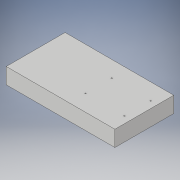
# Autodesk Inventor part: Chassis
Saved by Autodesk Inventor 2019 (Build 230136000, 136)
## iProperties
Created: 2020-02-14
Part Number: Chassis
Material: Generic
Document SubType Name: Modeling
Designer: close
Density: 1 g/cm^3
Appearance: Default
Author: close
Autodesk Inventor part; units mm, degrees
ref_plane "YZ Plane" through (0, 0, 0) normal (1, 0, 0) x (0, 1, 0)
ref_plane "XZ Plane" through (0, 0, 0) normal (0, 1, 0) x (-1, 0, 0)
ref_plane "XY Plane" through (0, 0, 0) normal (0, 0, 1) x (1, 0, 0)
sketch "Sketch1" plane through (0, 0, 0) normal (0, 1, 0) x (-1, 0, 0)
  line L0 (0, 0) -> (240, 0)
  line L1 (240, 0) -> (240, -130)
  line L2 (240, -130) -> (0, -130)
  line L3 (0, -130) -> (0, 0)
  dimension "d0" = 130
  dimension "d1" = 240
  constraints: 8 end point, 2 parallel, 1 horizontal, 1 perpendicular
  measures "d0" distance between parallel lines of L2 L0
  measures "d1" distance between parallel lines of L3 L1
extrude "Extrusion1" add sketch "Sketch1" along normal blind 35
sketch "Sketch2" plane through (0, 0, 0) normal (0, -1, 0) x (1, 0, 0)
  line L0 (-5, -111) -> (-105, -111) construction
  line L1 (-105, -111) -> (-105, -32) construction
  line L2 (-105, -32) -> (-5, -32) construction
  line L3 (-5, -32) -> (-5, -111) construction
  line L4 (-15, -94) -> (-101, -94) construction
  line L5 (-101, -94) -> (-101, -36) construction
  line L6 (-101, -36) -> (-15, -36) construction
  line L7 (-15, -36) -> (-15, -94) construction
  line L8 (-103.25, -76.2) -> (-99.35, -76.2) construction
  line L9 (-99.35, -76.2) -> (-99.35, -53.8) construction
  line L10 (-99.35, -53.8) -> (-103.25, -53.8) construction
  line L11 (-103.25, -53.8) -> (-103.25, -76.2) construction
  line L12 (0, 0) -> (-240, 0) construction
  line L13 (-240, -130) -> (0, -130) construction
  line L14 (-2.5, -113.5) -> (-107.5, -113.5)
  line L15 (-107.5, -113.5) -> (-107.5, -29.5)
  line L16 (-107.5, -29.5) -> (-2.5, -29.5)
  line L17 (-2.5, -29.5) -> (-2.5, -113.5)
  line L18 (0, -130) -> (0, 0) projected
  dimension "d5" = 100
  dimension "d6" = 86
  dimension "d7" = 58
  dimension "d8" = 79
  dimension "d9" = 4
  dimension "d10" = 4
  dimension "d12" = 22.4
  dimension "d13" = 17.8
  dimension "d14" = 130
  dimension "d16" = 53.8
  dimension "d17" = 3.9
  dimension "d18" = 1.75
  dimension "d19" = 105
  dimension "d20" = 2.5
  dimension "d21" = 84
  dimension "d22" = 2.5
  dimension "d25" = 2.5
  constraints: 32 end point, 8 parallel, 4 horizontal, 4 perpendicular
  measures "d5" distance of L0.start L0.end
  measures "d6" distance of L4.start L4.end
  measures "d7" distance of L6.end L4.start
  measures "d8" distance of L2.end L0.start
  measures "d9" distance between parallel lines of L2 L6
  measures "d10" distance between parallel lines of L1 L5
  measures "d12" distance between parallel lines of L10 L8
  measures "d13" distance from line of L5.end L10
  measures "d14" distance between parallel lines of L12 L13
  measures "d16" distance between parallel lines of L13 L8
  measures "d17" distance between parallel lines of L11 L9
  measures "d18" distance between parallel lines of L1 L11
  measures "d19" distance of L14.start L14.end
  measures "d20" distance between parallel lines of L18 L17
  measures "d21" distance between parallel lines of L16 L14
  measures "d22" distance between parallel lines of L0 L14
  measures "d25" distance between parallel lines of L17 L3
extrude "Extrusion2" cut sketch "Sketch2" against normal blind 32.5
sketch "Sketch3" plane through (0, 32.5, 0) normal (0, -1, 0) x (1, 0, 0)
  circle A0 centre (-15, -94) radius 3
  circle A1 centre (-101, -94) radius 3
  circle A2 centre (-15, -36) radius 3
  circle A3 centre (-101, -36) radius 3
  point P0 (0, 0)
  dimension "d26" = 6
  dimension "d27" = 6
  dimension "d28" = 6
  dimension "d29" = 6
  constraints: 4 centre point, 4 coincident
  measures "d26" diameter of A0
  measures "d27" diameter of A1
  measures "d28" diameter of A2
  measures "d29" diameter of A3
extrude "Extrusion3" add sketch "Sketch3" along normal blind 1.5
fillet "Fillet1" radius 1 4 edges at (-18, 32.5, -94) (-104, 32.5, -94) (-18, 32.5, -36) (-104, 32.5, -36)
sketch "Sketch4" plane through (-15, 31, -94) normal (0, -1, 0) x (1, 0, 0)
  circle A0 centre (0, 0) radius 3 construction
  circle A1 centre (0, 58) radius 3 construction
  circle A2 centre (-86, 58) radius 3 construction
  circle A3 centre (-86, 0) radius 3 construction
  circle A4 centre (0, 0) radius 3 construction
  circle A5 centre (-86, 58) radius 4 construction
  point P0 (15, 94)
  constraints: 4 coincident
hole "Hole1" at (-15, 31, -94) at (-15, 31, -36) at (-101, 31, -36) at (-101, 31, -94) direction (0, 1, 0) diameter 2.4 depth 4
equation "\"d10\" = d9"
equation "\"d16\" = -0.5 * d12 + 0.5 * d14"
equation "\"d22\" = -0.5 * d8 + 0.5 * d21"
equation "\"d25\" = -0.5 * d5 + 0.5 * d19"
body "Solid1"
